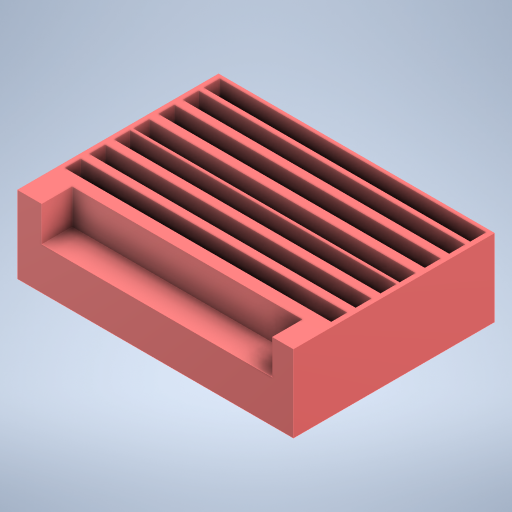
# Autodesk Inventor part: Motor_vez
Saved by Autodesk Inventor 2023 (Build 270158000, 158)
## iProperties
Created: 2023-04-27
Part Number: Motor_vez
Material: Generic
Document SubType Name: Modeling
Designer: nagyb
Density: 1 g/cm^3
Appearance: Smooth - Red
Author: nagyb
Autodesk Inventor part; units mm, degrees
ref_plane "YZ Plane" through (0, 0, 0) normal (1, 0, 0) x (0, 1, 0)
ref_plane "XZ Plane" through (0, 0, 0) normal (0, 1, 0) x (-1, 0, 0)
ref_plane "XY Plane" through (0, 0, 0) normal (0, 0, 1) x (1, 0, 0)
sketch "Sketch1" plane through (0, 0, 0) normal (0, 1, 0) x (-1, 0, 0)
  line L0 (-59, -43) -> (59, -43)
  line L1 (59, -43) -> (59, 43)
  line L2 (59, 43) -> (-59, 43)
  line L3 (-59, 43) -> (-59, -43)
  line L4 (-59, -43) -> (59, 43) construction
  line L5 (59, -43) -> (-59, 43) construction
  line L6 (56.9723, 41.5222) -> (-57.0608, 41.5222)
  line L7 (-57.0608, 41.5222) -> (-57.0608, 34.6385)
  line L8 (-57.0608, 34.6385) -> (56.9723, 34.6385)
  line L9 (56.9723, 34.6385) -> (56.9723, 41.5222)
  line L10 (56.9723, 32.5324) -> (-57.0608, 32.5324)
  line L11 (-57.0608, 32.5324) -> (-57.0608, 25.6486)
  line L12 (-57.0608, 25.6486) -> (56.9723, 25.6486)
  line L13 (56.9723, 25.6486) -> (56.9723, 32.5324)
  line L14 (56.9723, 22.0925) -> (-57.0608, 22.0925)
  line L15 (-57.0608, 22.0925) -> (-57.0608, 15.2088)
  line L16 (-57.0608, 15.2088) -> (56.9723, 15.2088)
  line L17 (56.9723, 15.2088) -> (56.9723, 22.0925)
  line L18 (56.9723, 11.3627) -> (-57.0608, 11.3627)
  line L19 (-57.0608, 11.3627) -> (-57.0608, 4.479)
  line L20 (-57.0608, 4.479) -> (56.9723, 4.479)
  line L21 (56.9723, 4.479) -> (56.9723, 11.3627)
  line L22 (56.9723, 3.1636) -> (-57.0608, 3.1636)
  line L23 (-57.0608, 3.1636) -> (-57.0608, -3.7202)
  line L24 (-57.0608, -3.7202) -> (56.9723, -3.7202)
  line L25 (56.9723, -3.7202) -> (56.9723, 3.1636)
  line L26 (56.9723, -7.487) -> (-57.0608, -7.487)
  line L27 (-57.0608, -7.487) -> (-57.0608, -14.3707)
  line L28 (-57.0608, -14.3707) -> (56.9723, -14.3707)
  line L29 (56.9723, -14.3707) -> (56.9723, -7.487)
  line L30 (56.9723, -17.9268) -> (-57.0608, -17.9268)
  line L31 (-57.0608, -17.9268) -> (-57.0608, -24.8106)
  line L32 (-57.0608, -24.8106) -> (56.9723, -24.8106)
  line L33 (56.9723, -24.8106) -> (56.9723, -17.9268)
  line L34 (49.9475, -43) -> (-48.6509, -43)
  line L35 (-48.6509, -43) -> (-48.6509, -30.0305)
  line L36 (-48.6509, -30.0305) -> (49.9475, -30.0305)
  line L37 (49.9475, -30.0305) -> (49.9475, -43)
  point P0 (0, 0)
  dimension "d0" = 118
  dimension "d1" = 86
  constraints: 76 end point, 18 parallel, 9 horizontal, 9 perpendicular, 2 midpoint, 2 point on line
  measures "d0" distance of L1.end L2.end
  measures "d1" distance of L0.end L1.end
extrude "Extrusion1" add sketch "Sketch1" along normal blind 33 contours L3 L2 L1 L0 L37 L36 L35 | L35 L36 L37 L0 | L9 L8 L7 L6 | L13 L12 L11 L10 | L17 L16 L15 L14 | L21 L20 L19 L18 | L25 L24 L23 L22 | L29 L28 L27 L26 | L33 L32 L31 L30
sketch "Sketch2" plane through (0, 33, 0) normal (0, 1, 0) x (1, 0, 0)
  line L0 (-59, -43) -> (59, -43)
  line L1 (59, -43) -> (59, 43)
  line L2 (59, 43) -> (-59, 43)
  line L3 (-59, 43) -> (-59, -43)
  line L4 (-59, -43) -> (59, 43) construction
  line L5 (59, -43) -> (-59, 43) construction
  line L6 (56.9723, 41.5222) -> (-57.0608, 41.5222)
  line L7 (-57.0608, 41.5222) -> (-57.0608, 34.6385)
  line L8 (-57.0608, 34.6385) -> (56.9723, 34.6385)
  line L9 (56.9723, 34.6385) -> (56.9723, 41.5222)
  line L10 (56.9723, 25.6486) -> (56.9723, 32.5324)
  line L11 (-57.0608, 25.6486) -> (56.9723, 25.6486)
  line L12 (56.9723, 32.5324) -> (-57.0608, 32.5324)
  line L13 (-57.0608, 32.5324) -> (-57.0608, 25.6486)
  line L14 (56.9723, 15.2088) -> (56.9723, 22.0925)
  line L15 (-57.0608, 15.2088) -> (56.9723, 15.2088)
  line L16 (56.9723, 22.0925) -> (-57.0608, 22.0925)
  line L17 (-57.0608, 22.0925) -> (-57.0608, 15.2088)
  line L18 (56.9723, 4.479) -> (56.9723, 11.3627)
  line L19 (-57.0608, 4.479) -> (56.9723, 4.479)
  line L20 (56.9723, 11.3627) -> (-57.0608, 11.3627)
  line L21 (-57.0608, 11.3627) -> (-57.0608, 4.479)
  line L22 (56.9723, -3.7202) -> (56.9723, 3.1636)
  line L23 (-57.0608, -3.7202) -> (56.9723, -3.7202)
  line L24 (56.9723, 3.1636) -> (-57.0608, 3.1636)
  line L25 (-57.0608, 3.1636) -> (-57.0608, -3.7202)
  line L26 (56.9723, -14.3707) -> (56.9723, -7.487)
  line L27 (-57.0608, -14.3707) -> (56.9723, -14.3707)
  line L28 (56.9723, -7.487) -> (-57.0608, -7.487)
  line L29 (-57.0608, -7.487) -> (-57.0608, -14.3707)
  line L30 (56.9723, -24.8106) -> (56.9723, -17.9268)
  line L31 (-57.0608, -24.8106) -> (56.9723, -24.8106)
  line L32 (56.9723, -17.9268) -> (-57.0608, -17.9268)
  line L33 (-57.0608, -17.9268) -> (-57.0608, -24.8106)
  line L34 (49.9475, -43) -> (-48.6509, -43)
  line L35 (-48.6509, -43) -> (-48.6509, -30.0305)
  line L36 (-48.6509, -30.0305) -> (49.9475, -30.0305)
  line L37 (49.9475, -30.0305) -> (49.9475, -43)
  point P0 (0, 0)
  point P1 (0, 0)
  dimension "d4" = 118
  dimension "d5" = 86
  constraints: 76 end point, 18 parallel, 9 horizontal, 9 perpendicular, 2 midpoint, 2 point on line
  measures "d4" distance of L1.end L5.end
  measures "d5" distance of L1.start L1.end
extrude "Extrusion2" cut sketch "Sketch2" against normal blind 15 contours L35 L36 L37 L0 | L9 L8 L7 L6 | L11 L13 L12 L10 | L15 L17 L16 L14 | L19 L21 L20 L18 | L23 L25 L24 L22 | L27 L29 L28 L26 | L31 L33 L32 L30
body "Solid1"
